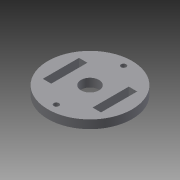
# Autodesk Inventor part: arm-servo
Saved by Autodesk Inventor 2013 (Build 170138000, 138)
## iProperties
Created: 2012-09-08
Part Number: arm-servo
Material: Generic
Document SubType Name: Modeling
Designer: frankenteddy
Density: 1 g/cm^3
Author: frankenteddy
Autodesk Inventor part; units mm, degrees
ref_plane "YZ Plane" through (0, 0, 0) normal (1, 0, 0) x (0, 1, 0)
ref_plane "XZ Plane" through (0, 0, 0) normal (0, 1, 0) x (-1, 0, 0)
ref_plane "XY Plane" through (0, 0, 0) normal (0, 0, 1) x (1, 0, 0)
sketch "Block1" plane through (0, 0, 0) normal (0, 0, 1) x (1, 0, 0)
  circle A0 centre (74.029, 24.2723) radius 1
  line L0 (49.279, 30.4723) -> (71.779, 30.4723)
  line L1 (71.779, 30.4723) -> (71.779, 18.0723)
  line L2 (71.779, 18.0723) -> (49.279, 18.0723)
  line L3 (49.279, 18.0723) -> (49.279, 30.4723)
  line L4 (49.279, 30.4723) -> (44.779, 30.4723)
  line L5 (44.779, 30.4723) -> (44.779, 18.0723)
  line L6 (44.779, 18.0723) -> (49.279, 18.0723)
  line L7 (49.279, 18.0723) -> (49.279, 30.4723)
  line L8 (71.779, 30.4723) -> (76.279, 30.4723)
  line L9 (76.279, 30.4723) -> (76.279, 18.0723)
  line L10 (76.279, 18.0723) -> (71.779, 18.0723)
  line L11 (71.779, 18.0723) -> (71.779, 30.4723)
  line L12 (44.779, 24.2723) -> (76.279, 24.2723) construction
  line L13 (47.029, 30.4723) -> (47.029, 18.0723) construction
  circle A1 centre (47.029, 24.2723) radius 1
  line L14 (74.029, 30.4723) -> (74.029, 18.0723) construction
  point P0 (60.979, 24.0984)
  dimension "d7" = 22.5
  dimension "d8" = 12.4
  dimension "d9" = 4.5
  dimension "d10" = 4.5
  dimension "d11" = 2
  dimension "d12" = 2
  measures "d7" distance of L1.end L2.end
  measures "d8" distance of L0.end L1.end
  measures "d9" distance of L6.end L5.end
  measures "d10" distance of L9.end L10.end
  measures "d11" diameter of A0
  measures "d12" diameter of A1
sketch "Sketch1" plane through (0, 0, 0) normal (0, 0, 1) x (1, 0, 0)
  line L0 (-92.7646, -8.503) -> (-89.7646, -8.503)
  line L1 (-89.7646, -8.503) -> (-89.7646, -11.753)
  line L2 (-89.7646, -11.753) -> (-92.7646, -11.753)
  line L3 (-92.7646, -11.753) -> (-92.7646, -8.503)
  line L4 (-92.7646, -21.6527) -> (-89.7646, -21.6527)
  line L5 (-89.7646, -21.6527) -> (-89.7646, -21.7527)
  line L6 (-89.7646, -21.7527) -> (-92.7646, -21.7527)
  line L7 (-92.7646, -21.7527) -> (-92.7646, -21.6527)
  circle A0 centre (0, 0) radius 16.25
  circle A1 centre (0, 13) radius 1
  line L8 (-16.25, 0) -> (16.25, 0) construction
  line L9 (0, 16.25) -> (0, -16.25) construction
  circle A2 centre (0, -13) radius 1
  circle A3 centre (0, 0) radius 3.5
  line L10 (-11.25, 7) -> (-8, 7)
  line L11 (-8, 7) -> (-8, -7)
  line L12 (-8, -7) -> (-11.25, -7)
  line L13 (-11.25, -7) -> (-11.25, 7)
  line L14 (-11.25, 0) -> (-8, 0) construction
  line L15 (11.25, 7) -> (8, 7)
  line L16 (8, 7) -> (8, -7)
  line L17 (8, -7) -> (11.25, -7)
  line L18 (11.25, -7) -> (11.25, 7)
  line L19 (11.25, 0) -> (8, 0) construction
  dimension "d0" = 3
  dimension "mat" = 3.25
  dimension "d2" = 3
  dimension "d3" = 0.1
  dimension "d23" = 32.5
  dimension "d24" = 2
  dimension "d25" = 12
  dimension "d28" = 7
  dimension "d29" = 3.25
  dimension "d30" = 14
  dimension "d31" = 5
  constraints: 40 end point, 7 parallel, 7 symmetric about line, 4 centre point, 4 perpendicular, 4 point on circle, 3 horizontal, 2 coincident, 2 midpoint, 1 collinear, 1 point on line, 1 other
  measures "d0" distance of L1.end L3.start
  measures "mat" distance of L1.start L1.end
  measures "d2" distance of L5.end L7.start
  measures "d3" distance of L5.start L5.end
  measures "d23" diameter of A0
  measures "d24" diameter of A1
  measures "d25" distance edge to line of A1 L8
  measures "d28" diameter of A3
  measures "d29" distance of L11.end L12.end
  measures "d30" distance of L10.end L11.end
  measures "d31" distance edge to line of A0 L13
extrude "Extrusion3" add sketch "Sketch1" along normal blind 3.25 contours A0
equation "\"d29\" = mat"
equation "\"d32\" = mat"
body "Solid3"
